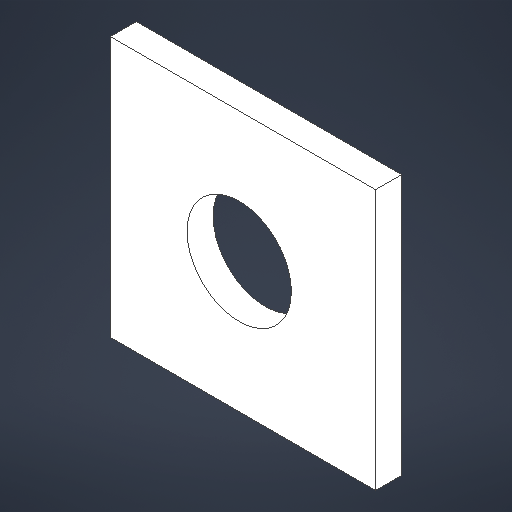
# Autodesk Inventor part: Top Connecter 1-
Saved by Autodesk Inventor 2026.1 (Build 301233020, 233B)
## iProperties
Created: 2025-11-30
Part Number: Top Connecter 1-
Material: Generic
Document SubType Name: Modeling
Designer: sarab
Density: 1 g/cm^3
Appearance: Default
Author: sarab
Autodesk Inventor part; units mm, degrees
ref_plane "YZ Plane" through (0, 0, 0) normal (1, 0, 0) x (0, 1, 0)
ref_plane "XZ Plane" through (0, 0, 0) normal (0, 1, 0) x (-1, 0, 0)
ref_plane "XY Plane" through (0, 0, 0) normal (0, 0, 1) x (1, 0, 0)
sketch "Sketch1" plane through (0, 0, 0) normal (0, 0, 1) x (1, 0, 0)
  line L0 (57.8123, 10.9423) -> (57.8123, -38.9997)
  line L1 (57.8123, -38.9997) -> (18.5273, -38.9997)
  circle A0 centre (31.6703, -14.0287) radius 10
  line L2 (18.5273, 10.9423) -> (57.8123, 10.9423)
  line L3 (18.5273, 10.9423) -> (12.7453, 10.9423)
  line L4 (12.7453, -38.9997) -> (18.5273, -38.9997)
  line L5 (12.7453, 10.9423) -> (6.9678, 10.9423)
  line L6 (6.9678, 10.9423) -> (6.9678, -38.9997)
  line L7 (6.9678, -38.9997) -> (12.7453, -38.9997)
  point P0 (0, 0)
  constraints: 16 end point, 4 perpendicular, 3 horizontal, 1 centre point
extrude "Extrusion1" add sketch "Sketch1" along normal blind 5
body "Solid1"
